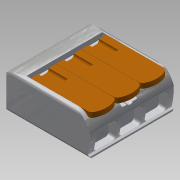
# Autodesk Inventor part: 221-413
Saved by Autodesk Inventor 2020.1 (Build 241239000, 239)
## iProperties
Created: 2019-12-10
Part Number: 221-413
Catalog Web Link: https://www.wago.com/us/wire-splicing-connectors/compact-splicing-connector/p/221-413
Description: 221-413-COMPACT splicing connectors for all conductor types 3-conductor terminal block
Vendor: WAGO
Document SubType Name: Modeling
Designer: Autodesk Inc.
Manufacturer: WAGO
Mass: 2.46 g
Surface Area: 17.0313 cm^2
Volume: 2.59959 cm^3
Density: 1 g/cm^3
Material: Generic
Appearance: PSOLRGB-175-175-175
Category: FIRST Choice
Company: Autodesk Inc.
PSOL_IDENT_0: {$CADENAS_DATA\23d-libs\wago\pg07\serie221\0221-0413_0999-0962.prj},157 {VTYP=3D},{NB=221-413},{LINA=
PSOL_IDENT_1: 221-413},{NN=221-413},{DATE=29.09.2017 05:32:44},{GEOMDATE=20.05.2014 11:52:00},{VERSION=},{LINEID=2
PSOL_IDENT_2: 0},{LINESUBID=-1},{WBVAR=}  {NB=221-413},{LINA=221-413},{KT=DUMMY},{BESTNR=221-413},{INFODE=Info DE}
PSOL_IDENT_3: ,{INFOEN=Info EN},{QUERSCHNITT1=0.2 - 4 \"e + m\"  /  0.14 - 4 \"f\"},{QUERSCHNITT2=24 - 12},{ABISOL
PSOL_IDENT_4: IERLAENGE=11},{SPANNUNG=450},{BEMESSSTOSSSPG=4},{VERSCHMUTZGRAD=2},{STROM=32},{P=3},{HOEHE=8.30},{BR
PSOL_IDENT_5: EITE=18.70},{TIEFE=18.60},{ANZAHLKLEMMSTEL=3},{ANZAHLPOTENTIAL=3},{FARBE=transparent},{GEWICHT=2.460
PSOL_IDENT_6: },{LINKDE=http://eshop.wago.com},{LINKEN=http://eshop.wago.com}
NN: 221-413
NT: COMPACT splicing connectors for all conductor types 3-conductor terminal block
NB: 221-413
NBSYN: $BESTNR.
LINA: 221-413
OFFICIAL_STANDARD_NUMBERS: NO
BESTNR: 221-413
INFODE: Info DE
INFOEN: Info EN
QUERSCHNITT1: 0.2 - 4 "e + m"  /  0.14 - 4 "f"
QUERSCHNITT2: 24 - 12
ABISOLIERLAENGE: 11
SPANNUNG: 450
BEMESSSTOSSSPG: 4
VERSCHMUTZGRAD: 2
STROM: 32
P: 3
HOEHE: 8.30
BREITE: 18.70
TIEFE: 18.60
ANZAHLKLEMMSTEL: 3
ANZAHLPOTENTIAL: 3
FARBE: transparent
GEWICHT: 2.460
SUPPLIER: WAGO
ARTICLENO: 221-413
BOMINFO: 221-413
CREATOR: CADENAS GmbH
Author: Autodesk Inc.
Comments: COMPACT splicing connectors for all conductor types 3-conductor terminal block
Autodesk Inventor part; units mm, degrees
ref_plane "YZ Plane" through (0, 0, 0) normal (1, 0, 0) x (0, 1, 0)
ref_plane "XZ Plane" through (0, 0, 0) normal (0, 1, 0) x (-1, 0, 0)
ref_plane "XY Plane" through (0, 0, 0) normal (0, 0, 1) x (1, 0, 0)
sketch "Sketch_1" plane through (0, 0, 0) normal (0, 0, 1) x (1, 0, 0)
  line L0 (0, 7.2187) -> (0, 0)
  line L1 (0, 0) -> (18.4, 0)
  arc A0 (18.4, 0) -> (18.6, 0.2) centre (18.4, 0.2) ccw
  line L2 (18.6, 0.2) -> (18.6, 0.2905)
  arc A1 (18.6, 0.2905) -> (18.4845, 0.4717) centre (18.4, 0.2905) ccw
  line L3 (18.4845, 0.4717) -> (18.1022, 0.65)
  arc A2 (18.1022, 0.65) -> (18.5749, 4.9468) centre (4.69, 4.3) ccw
  arc A3 (18.5749, 4.9468) -> (18.4726, 5.3431) centre (17.576, 4.9002) ccw
  arc A4 (18.4726, 5.3431) -> (17.0892, 7.3213) centre (11.3, 1.8) ccw
  arc A5 (17.0892, 7.3213) -> (15.23, 8.15) centre (15.23, 5.65) ccw
  line L4 (15.23, 8.15) -> (3.62, 8.15)
  arc A6 (3.62, 8.15) -> (0.3643, 7.6999) centre (3.62, -3.85) ccw
  arc A7 (0.3643, 7.6999) -> (0, 7.2187) centre (0.5, 7.2187) ccw
  constraints: 16 point on circle, 10 end point, 8 centre point
extrude "Extrusion1" add sketch "Sketch_1" along normal blind 18.6
sketch "Sketch_5" plane through (0, 0, 0) normal (1, 0, 0) x (0, 1, 0)
  line L0 (9.15, 19.6) -> (-1, 19.6)
  line L1 (-1, 19.6) -> (-1, -1)
  line L2 (-1, -1) -> (9.15, -1)
  line L3 (9.15, -1) -> (9.15, 19.6)
  line L4 (7.45, 18.6) -> (0.7, 18.6)
  arc A0 (0.7, 18.6) -> (0, 17.9) centre (0.7, 17.9) ccw
  line L5 (0, 17.9) -> (0, 0.7)
  arc A1 (0, 0.7) -> (0.7, 0) centre (0.7, 0.7) ccw
  line L6 (0.7, 0) -> (7.45, 0)
  arc A2 (7.45, 0) -> (8.15, 0.7) centre (7.45, 0.7) ccw
  line L7 (8.15, 0.7) -> (8.15, 17.9)
  arc A3 (8.15, 17.9) -> (7.45, 18.6) centre (7.45, 17.9) ccw
  constraints: 16 end point, 8 point on circle, 4 centre point
extrude "Extrusion2" cut sketch "Sketch_5" along normal blind 18.6
sketch "Sketch_2" plane through (18.6, 0, 0) normal (1, 0, 0) x (0, 0, -1)
  line L0 (-6.15, 4.07) -> (-6.15, 1.35)
  arc A0 (-6.15, 1.35) -> (-5.45, 0.65) centre (-5.45, 1.35) ccw
  line L1 (-5.45, 0.65) -> (-1.95, 0.65)
  arc A1 (-1.95, 0.65) -> (-1.25, 1.35) centre (-1.95, 1.35) ccw
  line L2 (-1.25, 1.35) -> (-1.25, 4.07)
  arc A2 (-1.25, 4.07) -> (-1.95, 4.77) centre (-1.95, 4.07) ccw
  line L3 (-1.95, 4.77) -> (-5.45, 4.77)
  arc A3 (-5.45, 4.77) -> (-6.15, 4.07) centre (-5.45, 4.07) ccw
  constraints: 8 end point, 8 point on circle, 4 centre point
extrude "Extrusion3" cut sketch "Sketch_2" against normal blind 2
sketch "Pattern_1_SKETCH_1" plane through (18.6, 0, 0) normal (1, 0, 0) x (0, 0, -1)
  line L0 (-11.75, 4.07) -> (-11.75, 1.35)
  arc A0 (-11.75, 1.35) -> (-11.05, 0.65) centre (-11.05, 1.35) ccw
  line L1 (-11.05, 0.65) -> (-7.55, 0.65)
  arc A1 (-7.55, 0.65) -> (-6.85, 1.35) centre (-7.55, 1.35) ccw
  line L2 (-6.85, 1.35) -> (-6.85, 4.07)
  arc A2 (-6.85, 4.07) -> (-7.55, 4.77) centre (-7.55, 4.07) ccw
  line L3 (-7.55, 4.77) -> (-11.05, 4.77)
  arc A3 (-11.05, 4.77) -> (-11.75, 4.07) centre (-11.05, 4.07) ccw
  constraints: 8 end point, 8 point on circle, 4 centre point
sketch "Pattern_1_SKETCH_2" plane through (18.6, 0, 0) normal (1, 0, 0) x (0, 0, -1)
  line L0 (-17.35, 4.07) -> (-17.35, 1.35)
  arc A0 (-17.35, 1.35) -> (-16.65, 0.65) centre (-16.65, 1.35) ccw
  line L1 (-16.65, 0.65) -> (-13.15, 0.65)
  arc A1 (-13.15, 0.65) -> (-12.45, 1.35) centre (-13.15, 1.35) ccw
  line L2 (-12.45, 1.35) -> (-12.45, 4.07)
  arc A2 (-12.45, 4.07) -> (-13.15, 4.77) centre (-13.15, 4.07) ccw
  line L3 (-13.15, 4.77) -> (-16.65, 4.77)
  arc A3 (-16.65, 4.77) -> (-17.35, 4.07) centre (-16.65, 4.07) ccw
  constraints: 8 end point, 8 point on circle, 4 centre point
extrude "Extrusion4" cut sketch "Pattern_1_SKETCH_1" against normal blind 2
extrude "Extrusion5" cut sketch "Pattern_1_SKETCH_2" against normal blind 2
sketch "Sketch_4" plane through (18.6, 0, 0) normal (1, 0, 0) x (0, 0, -1)
  line L0 (-11.075, 7.3) -> (-11.075, 6.3)
  arc A0 (-11.075, 6.3) -> (-10.775, 6) centre (-10.775, 6.3) ccw
  line L1 (-10.775, 6) -> (-9.9408, 6)
  arc A1 (-9.9408, 6) -> (-8.6592, 6) centre (-9.3, 6.8) ccw
  line L2 (-8.6592, 6) -> (-7.825, 6)
  arc A2 (-7.825, 6) -> (-7.525, 6.3) centre (-7.825, 6.3) ccw
  line L3 (-7.525, 6.3) -> (-7.525, 7.3)
  arc A3 (-7.525, 7.3) -> (-7.825, 7.6) centre (-7.825, 7.3) ccw
  line L4 (-7.825, 7.6) -> (-8.6592, 7.6)
  arc A4 (-8.6592, 7.6) -> (-9.9408, 7.6) centre (-9.3, 6.8) ccw
  line L5 (-9.9408, 7.6) -> (-10.775, 7.6)
  arc A5 (-10.775, 7.6) -> (-11.075, 7.3) centre (-10.775, 7.3) ccw
  constraints: 12 end point, 12 point on circle, 6 centre point
extrude "Extrusion6" cut sketch "Sketch_4" against normal blind 2
sketch "Sketch_6" plane through (18.6, 0, 0) normal (1, 0, 0) x (0, 0, -1)
  line L0 (-6.5, 7) -> (-5.96, 7)
  line L1 (-5.96, 7) -> (-5.96, 8.15)
  line L2 (-5.96, 8.15) -> (-1.44, 8.15)
  line L3 (-1.44, 8.15) -> (-1.44, 7)
  line L4 (-1.44, 7) -> (-0.9, 7)
  line L5 (-0.9, 7) -> (-0.9, 9.15)
  line L6 (-0.9, 9.15) -> (-6.5, 9.15)
  line L7 (-6.5, 9.15) -> (-6.5, 7)
  constraints: 16 end point
extrude "Extrusion7" cut sketch "Sketch_6" against normal blind 14.98
sketch "Pattern_2_SKETCH_1" plane through (18.6, 0, 0) normal (1, 0, 0) x (0, 0, -1)
  line L0 (-17.7, 7) -> (-17.16, 7)
  line L1 (-17.16, 7) -> (-17.16, 8.15)
  line L2 (-17.16, 8.15) -> (-12.64, 8.15)
  line L3 (-12.64, 8.15) -> (-12.64, 7)
  line L4 (-12.64, 7) -> (-12.1, 7)
  line L5 (-12.1, 7) -> (-12.1, 9.15)
  line L6 (-12.1, 9.15) -> (-17.7, 9.15)
  line L7 (-17.7, 9.15) -> (-17.7, 7)
  constraints: 16 end point
extrude "Extrusion8" cut sketch "Pattern_2_SKETCH_1" against normal blind 14.98
sketch "Sketch_13" plane through (18.6, 0, 0) normal (1, 0, 0) x (0, 0, -1)
  line L0 (-12.1, 7) -> (-11.56, 7)
  line L1 (-11.56, 7) -> (-11.56, 8.15)
  line L2 (-11.56, 8.15) -> (-7.04, 8.15)
  line L3 (-7.04, 8.15) -> (-7.04, 7)
  line L4 (-7.04, 7) -> (-6.5, 7)
  line L5 (-6.5, 7) -> (-6.5, 9.15)
  line L6 (-6.5, 9.15) -> (-12.1, 9.15)
  line L7 (-12.1, 9.15) -> (-12.1, 7)
  constraints: 16 end point
extrude "Extrusion9" cut sketch "Sketch_13" against normal blind 14.98
sketch "Sketch_8" plane through (0, 8.15, 0) normal (0, 1, 0) x (1, 0, 0)
  line L0 (4.55, -5.98) -> (4.55, -6.48)
  line L1 (4.55, -6.48) -> (17.1821, -6.48)
  arc A0 (17.1821, -6.48) -> (18.0777, -5.925) centre (17.1821, -5.48) ccw
  arc A1 (18.0777, -5.925) -> (18.0777, -1.475) centre (13.6, -3.7) ccw
  arc A2 (18.0777, -1.475) -> (17.1821, -0.92) centre (17.1821, -1.92) ccw
  line L2 (17.1821, -0.92) -> (4.55, -0.92)
  line L3 (4.55, -0.92) -> (4.55, -1.42)
  line L4 (4.55, -1.42) -> (10.25, -1.42)
  arc A3 (10.65, -1.82) -> (10.25, -1.42) centre (10.25, -1.82) ccw
  line L5 (10.65, -1.82) -> (10.65, -5.58)
  arc A4 (10.25, -5.98) -> (10.65, -5.58) centre (10.25, -5.58) ccw
  line L6 (10.25, -5.98) -> (4.55, -5.98)
  constraints: 14 end point, 10 point on circle, 5 centre point
extrude "Extrusion10" add sketch "Sketch_8" against normal blind 1.1
sketch "Pattern_3_SKETCH_1" plane through (0, 8.15, 0) normal (0, 1, 0) x (1, 0, 0)
  line L0 (4.55, -11.58) -> (4.55, -12.08)
  line L1 (4.55, -12.08) -> (17.1821, -12.08)
  arc A0 (17.1821, -12.08) -> (18.0777, -11.525) centre (17.1821, -11.08) ccw
  arc A1 (18.0777, -11.525) -> (18.0777, -7.075) centre (13.6, -9.3) ccw
  arc A2 (18.0777, -7.075) -> (17.1821, -6.52) centre (17.1821, -7.52) ccw
  line L2 (17.1821, -6.52) -> (4.55, -6.52)
  line L3 (4.55, -6.52) -> (4.55, -7.02)
  line L4 (4.55, -7.02) -> (10.25, -7.02)
  arc A3 (10.65, -7.42) -> (10.25, -7.02) centre (10.25, -7.42) ccw
  line L5 (10.65, -7.42) -> (10.65, -11.18)
  arc A4 (10.25, -11.58) -> (10.65, -11.18) centre (10.25, -11.18) ccw
  line L6 (10.25, -11.58) -> (4.55, -11.58)
  constraints: 14 end point, 10 point on circle, 5 centre point
sketch "Pattern_3_SKETCH_2" plane through (0, 8.15, 0) normal (0, 1, 0) x (1, 0, 0)
  line L0 (4.55, -17.18) -> (4.55, -17.68)
  line L1 (4.55, -17.68) -> (17.1821, -17.68)
  arc A0 (17.1821, -17.68) -> (18.0777, -17.125) centre (17.1821, -16.68) ccw
  arc A1 (18.0777, -17.125) -> (18.0777, -12.675) centre (13.6, -14.9) ccw
  arc A2 (18.0777, -12.675) -> (17.1821, -12.12) centre (17.1821, -13.12) ccw
  line L2 (17.1821, -12.12) -> (4.55, -12.12)
  line L3 (4.55, -12.12) -> (4.55, -12.62)
  line L4 (4.55, -12.62) -> (10.25, -12.62)
  arc A3 (10.65, -13.02) -> (10.25, -12.62) centre (10.25, -13.02) ccw
  line L5 (10.65, -13.02) -> (10.65, -16.78)
  arc A4 (10.25, -17.18) -> (10.65, -16.78) centre (10.25, -16.78) ccw
  line L6 (10.25, -17.18) -> (4.55, -17.18)
  constraints: 14 end point, 10 point on circle, 5 centre point
extrude "Extrusion11" add sketch "Pattern_3_SKETCH_1" against normal blind 1.1
extrude "Extrusion12" add sketch "Pattern_3_SKETCH_2" against normal blind 1.1
sketch "Sketch_10" plane through (3.62, 0, 0) normal (1, 0, 0) x (0, 0, -1)
  arc A0 (-4.86, 8) -> (-4.26, 7.4) centre (-4.26, 8) ccw
  line L0 (-4.26, 7.4) -> (-3.14, 7.4)
  arc A1 (-3.14, 7.4) -> (-2.54, 8) centre (-3.14, 8) ccw
  line L1 (-2.54, 8) -> (-2.54, 8.15)
  line L2 (-2.54, 8.15) -> (-4.86, 8.15)
  line L3 (-4.86, 8.15) -> (-4.86, 8)
  constraints: 8 end point, 4 point on circle, 2 centre point
extrude "Extrusion13" cut sketch "Sketch_10" along normal blind 5.2
sketch "Pattern_4_SKETCH_1" plane through (3.62, 0, 0) normal (1, 0, 0) x (0, 0, -1)
  arc A0 (-10.46, 8) -> (-9.86, 7.4) centre (-9.86, 8) ccw
  line L0 (-9.86, 7.4) -> (-8.74, 7.4)
  arc A1 (-8.74, 7.4) -> (-8.14, 8) centre (-8.74, 8) ccw
  line L1 (-8.14, 8) -> (-8.14, 8.15)
  line L2 (-8.14, 8.15) -> (-10.46, 8.15)
  line L3 (-10.46, 8.15) -> (-10.46, 8)
  constraints: 8 end point, 4 point on circle, 2 centre point
sketch "Pattern_4_SKETCH_2" plane through (3.62, 0, 0) normal (1, 0, 0) x (0, 0, -1)
  arc A0 (-16.06, 8) -> (-15.46, 7.4) centre (-15.46, 8) ccw
  line L0 (-15.46, 7.4) -> (-14.34, 7.4)
  arc A1 (-14.34, 7.4) -> (-13.74, 8) centre (-14.34, 8) ccw
  line L1 (-13.74, 8) -> (-13.74, 8.15)
  line L2 (-13.74, 8.15) -> (-16.06, 8.15)
  line L3 (-16.06, 8.15) -> (-16.06, 8)
  constraints: 8 end point, 4 point on circle, 2 centre point
extrude "Extrusion14" cut sketch "Pattern_4_SKETCH_1" along normal blind 5.2
extrude "Extrusion15" cut sketch "Pattern_4_SKETCH_2" along normal blind 5.2
sketch "Sketch_12" plane through (0, 0, 0.9) normal (0, 0, 1) x (1, 0, 0)
  line L0 (3.62, 7) -> (4.55, 7)
  line L1 (4.55, 7) -> (4.55, 8.15)
  line L2 (4.55, 8.15) -> (3.62, 8.15)
  line L3 (3.62, 8.15) -> (3.62, 7)
  constraints: 8 end point
extrude "Extrusion16" cut sketch "Sketch_12" along normal blind 16.8
body "Solid1"
